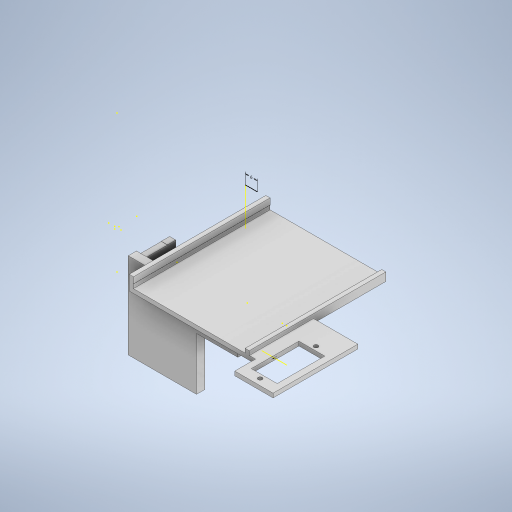
# Autodesk Inventor part: btholder
Saved by Autodesk Inventor 2023 (Build 270158000, 158)
## iProperties
Created: 2023-04-13
Part Number: btholder
Material: Generic
Document SubType Name: Modeling
Designer: Markus
Density: 1 g/cm^3
Appearance: Default
Author: Markus
Autodesk Inventor part; units mm, degrees
ref_plane "YZ Plane" through (0, 0, 0) normal (1, 0, 0) x (0, 1, 0)
ref_plane "XZ Plane" through (0, 0, 0) normal (0, 1, 0) x (-1, 0, 0)
ref_plane "XY Plane" through (0, 0, 0) normal (0, 0, 1) x (1, 0, 0)
sketch "Sketch1" plane through (0, 0, 0) normal (1, 0, 0) x (0, 1, 0)
  line L0 (0, 0) -> (20.5296, 0)
  line L1 (20.5296, -23) -> (0, -23)
  line L2 (0, -23) -> (0, 0)
  line L3 (0, 0) -> (50, 0)
  line L4 (50, 0) -> (50, -23)
  line L5 (50, -23) -> (0, -23)
  line L6 (0, -23) -> (0, 0)
  dimension "d0" = 23
  dimension "d1" = 50
  constraints: 14 end point, 3 parallel, 2 horizontal, 1 perpendicular, 1 point on line
  measures "d0" distance of L0.end L1.start
  measures "d1" distance of L4.end L5.end
extrude "Extrusion1" add sketch "Sketch1" along normal blind 2
sketch "Sketch2" plane through (2, 0, 0) normal (1, 0, 0) x (0, 0, -1)
  line L0 (23, 50) -> (0, 50) projected
  line L1 (13.5, 0) -> (9.5, 0)
  line L2 (9.5, 0) -> (9.5, 50)
  line L3 (9.5, 50) -> (13.5, 50)
  line L4 (13.5, 50) -> (13.5, 0)
  line L5 (13.5, 0) -> (9.5, 50) construction
  line L6 (9.5, 0) -> (13.5, 50) construction
  point P0 (0, 0)
  point P1 (17.2504, 25)
  point P2 (11.5, 25)
  dimension "d4" = 4
  constraints: 12 end point, 2 midpoint, 2 parallel, 1 horizontal, 1 perpendicular, 1 point on line
  measures "d4" distance of L2.end L3.end
sketch "Sketch3" plane through (0, 0, 0) normal (-1, 0, 0) x (0, 0, 1)
  line L0 (-23, 50) -> (0, 50) projected
  line L1 (-23, 50) -> (0, 50)
  line L2 (0, 50) -> (0, 0)
  line L3 (0, 0) -> (-23, 0)
  line L4 (-23, 0) -> (-23, 50)
  constraints: 8 end point, 2 parallel, 1 horizontal, 1 perpendicular
extrude "Extrusion2" add sketch "Sketch3" along normal blind 1
sketch "Sketch4" plane through (2, 0, 0) normal (1, 0, 0) x (0, 0, -1)
  point P0 (0, 0)
extrude "Extrusion3" add sketch "Sketch2" along normal blind 29
sketch "Sketch5" plane through (2, 0, -9.5) normal (0, 0, 1) x (1, 0, 0)
  line L0 (0, 50) -> (29, 50) projected
  line L1 (29, 0) -> (27, 0)
  line L2 (27, 0) -> (27, 50)
  line L3 (27, 50) -> (29, 50)
  line L4 (29, 50) -> (29, 0)
  point P0 (-2, 0)
  dimension "d9" = 2
  constraints: 8 end point, 2 parallel, 1 horizontal, 1 perpendicular, 1 point on line
  measures "d9" distance of L2.end L3.end
extrude "Extrusion4" add sketch "Sketch5" along normal blind 17.5
sketch "Sketch6" plane through (2, 0, -13.5) normal (0, 0, -1) x (-1, 0, 0)
  line L0 (-29, 50) -> (-27, 50) projected
  line L1 (-27, 50) -> (-27, 0) projected
  line L2 (-29, 50) -> (-27, 50)
  line L3 (-27, 50) -> (-27, 0)
  line L4 (-27, 0) -> (-29, 0)
  line L5 (-29, 0) -> (-29, 50)
  point P0 (2, 0)
  constraints: 8 end point, 2 parallel, 1 horizontal, 1 perpendicular
extrude "Extrusion5" add sketch "Sketch6" along normal blind 17.5
sketch "Sketch7" plane through (31, 0, 0) normal (1, 0, 0) x (0, 0, -1)
  line L0 (-8, 0) -> (-8, 50) projected
  line L1 (31, 50) -> (31, 0) projected
  line L2 (-8, 50) -> (31, 50)
  line L3 (31, 50) -> (31, 48)
  line L4 (31, 48) -> (-8, 48)
  line L5 (-8, 48) -> (-8, 50)
  point P0 (0, 0)
  dimension "d14" = 2
  constraints: 8 end point, 2 parallel, 1 horizontal, 1 perpendicular, 1 point on line
  measures "d14" distance of L2.end L3.end
extrude "Extrusion6" add sketch "Sketch7" along normal blind 32
sketch "Sketch8" plane through (31, 48, -31) normal (0, -1, 0) x (1, 0, 0)
  line L0 (32, 39) -> (32, 0) projected
  line L1 (0, 0) -> (32, 0) projected
  line L2 (32, 39) -> (30, 39)
  line L3 (30, 39) -> (30, 0)
  line L4 (30, 0) -> (32, 0)
  line L5 (32, 0) -> (32, 39)
  point P0 (-31, 31)
  dimension "d17" = 2
  constraints: 8 end point, 2 parallel, 1 horizontal, 1 perpendicular, 1 point on line
  measures "d17" distance of L4.end L3.end
extrude "Extrusion7" add sketch "Sketch8" along normal up to surface (48 mm away)
sketch "Sketch9" plane through (31, 48, -31) normal (0, -1, 0) x (1, 0, 0)
  point P0 (-31, 31)
sketch "Sketch10" plane through (61, 0, 8) normal (0, -1, 0) x (1, 0, 0)
  line L0 (2, -39) -> (2, 0) projected
  line L1 (-32, -17.5) -> (-32, 0) projected
  line L2 (2, 0) -> (-32, 0)
  line L3 (-32, 0) -> (-32, -9)
  line L4 (-32, -9) -> (2, -9)
  line L5 (2, -9) -> (2, 0)
  point P0 (-61, -8)
  dimension "d20" = 9
  constraints: 8 end point, 2 parallel, 1 horizontal, 1 perpendicular, 1 point on line
  measures "d20" distance of L3.end L2.end
extrude "Extrusion8" cut sketch "Sketch10" against normal blind 50
sketch "Sketch11" plane through (2, 0, -31) normal (0, 0, -1) x (-1, 0, 0)
  line L0 (-61, 50) -> (-61, 0) projected
  line L1 (0, 50) -> (-27, 50) projected
  line L2 (-61, 0) -> (-27, 0)
  line L3 (-27, 0) -> (-27, 50)
  line L4 (-27, 50) -> (-61, 50)
  line L5 (-61, 50) -> (-61, 0)
  point P0 (2, 0)
  constraints: 8 end point, 2 parallel, 1 horizontal, 1 perpendicular
extrude "Extrusion9" add sketch "Sketch11" along normal blind 2
sketch "Sketch12" plane through (-1, 0, 0) normal (0, -1, 0) x (1, 0, 0)
  line L0 (62, -1) -> (32, -1) projected
  line L1 (64, -1) -> (64, -33) projected
  line L2 (62, -1) -> (64, -1)
  line L3 (64, -1) -> (64, -31.0308)
  line L4 (64, -31.0308) -> (62, -31.0308)
  line L5 (62, -31.0308) -> (62, -1)
  point P0 (1, 0)
  constraints: 8 end point, 2 parallel, 1 horizontal, 1 perpendicular, 1 point on line
extrude "Extrusion10" add sketch "Sketch12" along normal blind 20.5
sketch "Sketch13" plane through (61, 48, -31) normal (-1, 0, 0) x (0, 0, 1)
  line L0 (30, -68.5) -> (-0.0308, -68.5) projected
  line L1 (30, 0) -> (30, -68.5) projected
  line L2 (-0.0308, -68.5) -> (30, -68.5)
  line L3 (30, -68.5) -> (30, -66.5)
  line L4 (30, -66.5) -> (-0.0308, -66.5)
  line L5 (-0.0308, -66.5) -> (-0.0308, -68.5)
  point P0 (31, -48)
  dimension "d27" = 2
  constraints: 8 end point, 2 parallel, 1 horizontal, 1 perpendicular, 1 point on line
  measures "d27" distance of L3.end L2.end
extrude "Extrusion11" add sketch "Sketch13" along normal up to surface (32 mm away)
sketch "Sketch14" plane through (-1, 0, 0) normal (0, -1, 0) x (1, 0, 0)
  line L0 (64, -33) -> (30, -33) projected
  line L1 (64, -31.0308) -> (30, -31.0308) projected
  line L2 (64, -33) -> (30, -33)
  line L3 (30, -33) -> (30, -31.0308)
  line L4 (30, -31.0308) -> (64, -31.0308)
  line L5 (64, -31.0308) -> (64, -33)
  point P0 (1, 0)
  point P1 (30, -33)
  constraints: 8 end point, 2 parallel, 1 horizontal, 1 perpendicular
extrude "Extrusion12" add sketch "Sketch14" along normal up to surface (20.5 mm away)
sketch "Sketch15" plane through (61, 48, -31) normal (-1, 0, 0) x (0, 0, 1)
  line L0 (-0.0308, -66.5) -> (30, -66.5) projected
  line L1 (30, 0) -> (30, -66.5) projected
  line L2 (-0.0308, -66.5) -> (30, -66.5)
  line L3 (30, -66.5) -> (30, -48)
  line L4 (30, -48) -> (-0.0308, -48)
  line L5 (-0.0308, -48) -> (-0.0308, -66.5)
  point P0 (31, -48)
  constraints: 8 end point, 2 parallel, 1 horizontal, 1 perpendicular, 1 point on line
extrude "Extrusion13" cut sketch "Sketch15" against normal blind 10
sketch "Sketch16" plane through (-1, 0, 0) normal (0, -1, 0) x (1, 0, 0)
  line L0 (32, -31) -> (32, -1) projected
  line L1 (30, -33) -> (64, -33) projected
  line L2 (32, -1) -> (30, -1)
  line L3 (30, -1) -> (30, -33)
  line L4 (30, -33) -> (32, -33)
  line L5 (32, -33) -> (32, -1)
  point P0 (1, 0)
  constraints: 8 end point, 2 parallel, 1 horizontal, 1 perpendicular
extrude "Extrusion14" add sketch "Sketch16" along normal up to surface (18.5 mm away)
sketch "Sketch17" plane through (31, 0, -31.0308) normal (0, 0, 1) x (1, 0, 0)
  line L0 (0, 48) -> (0, -18.5) projected
  line L1 (32, 50) -> (32, -20.5) projected
  line L2 (0, -18.5) -> (32, -18.5)
  line L3 (32, -18.5) -> (32, 0)
  line L4 (32, 0) -> (0, 0)
  line L5 (0, 0) -> (0, -18.5)
  point P0 (-31, 0)
  constraints: 8 end point, 2 parallel, 1 horizontal, 1 perpendicular, 1 point on line
extrude "Extrusion15" cut sketch "Sketch17" against normal blind 10
sketch "Sketch18" plane through (31, 0, 0) normal (1, 0, 0) x (0, 0, -1)
  line L0 (1, 48) -> (1, -18.5) projected
  line L1 (31, 0) -> (1, 0) projected
  line L2 (1, -18.5) -> (3, -18.5)
  line L3 (3, -18.5) -> (3, 0)
  line L4 (3, 0) -> (1, 0)
  line L5 (1, 0) -> (1, -18.5)
  point P0 (0, 0)
  dimension "d38" = 2
  constraints: 8 end point, 2 parallel, 1 horizontal, 1 perpendicular, 1 point on line
  measures "d38" distance of L4.end L3.end
extrude "Extrusion16" add sketch "Sketch18" along normal blind 13
sketch "Sketch19" plane through (29, 50, -1) normal (0, 0, 1) x (1, 0, 0)
  line L0 (34, -68.5) -> (34, -70.5) projected
  line L1 (34, -70.5) -> (0, -70.5) projected
  line L2 (34, -68.5) -> (0, -68.5)
  line L3 (0, -68.5) -> (0, -70.5)
  line L4 (0, -70.5) -> (34, -70.5)
  line L5 (34, -70.5) -> (34, -68.5)
  point P0 (-29, -50)
  constraints: 8 end point, 2 parallel, 1 horizontal, 1 perpendicular
extrude "Extrusion17" add sketch "Sketch19" along normal blind 2
sketch "Sketch20" plane through (31, -18.5, -33) normal (0, 1, 0) x (1, 0, 0)
  point P0 (-31, -33)
sketch "Sketch21" plane through (29, 50, -1) normal (0, 0, 1) x (1, 0, 0)
  line L0 (15, -50) -> (15, -68.5) projected
  line L1 (2, -68.5) -> (15, -68.5) projected
  line L2 (15, -50) -> (2, -50)
  line L3 (2, -50) -> (2, -68.5)
  line L4 (2, -68.5) -> (15, -68.5)
  line L5 (15, -68.5) -> (15, -50)
  point P0 (-29, -50)
  constraints: 8 end point, 2 parallel, 1 horizontal, 1 perpendicular
extrude "Extrusion18" cut sketch "Sketch21" against normal blind 2
sketch "Sketch22" plane through (31, -18.5, -33) normal (0, 1, 0) x (1, 0, 0)
  line L0 (32, -34) -> (-2, -34) projected
  line L1 (30, -32) -> (0, -32) projected
  line L2 (-2, -34) -> (13, -34)
  line L3 (13, -34) -> (13, -32)
  line L4 (13, -32) -> (-2, -32)
  line L5 (-2, -32) -> (-2, -34)
  point P0 (-31, -33)
  dimension "d45" = 15
  constraints: 8 end point, 2 parallel, 1 horizontal, 1 perpendicular, 1 point on line
  measures "d45" distance of L4.end L3.end
extrude "Extrusion19" add sketch "Sketch22" along normal blind 4
sketch "Sketch23" plane through (29, 50, 1) normal (0, 0, 1) x (1, 0, 0)
  point P0 (-29, -50)
sketch "Sketch24" plane through (63, 0, 0) normal (1, 0, 0) x (0, 0, -1)
  point P0 (0, 0)
sketch "Sketch25" plane through (63, 0, 0) normal (1, 0, 0) x (0, 0, -1)
  line L0 (-1, -20.5) -> (-1, -18.5) projected
  line L1 (33, -20.5) -> (-1, -20.5) projected
  line L2 (-1, -18.5) -> (33, -18.5)
  line L3 (33, -18.5) -> (33, -20.5)
  line L4 (33, -20.5) -> (-1, -20.5)
  line L5 (-1, -20.5) -> (-1, -18.5)
  point P0 (0, 0)
  constraints: 8 end point, 2 parallel, 1 horizontal, 1 perpendicular
extrude "Extrusion20" add sketch "Sketch25" along normal blind 5
sketch "Sketch26" plane through (68, 0, 0) normal (1, 0, 0) x (0, 0, -1)
  line L0 (1, -18.5) -> (33, -18.5) projected
  line L1 (33, -20.5) -> (-1, -20.5) projected
  line L2 (2.0812, -18.5) -> (-1, -18.5)
  line L3 (-1, -18.5) -> (-1, -20.5)
  line L4 (-1, -20.5) -> (2.0812, -20.5)
  line L5 (2.0812, -20.5) -> (2.0812, -18.5)
  point P0 (0, 0)
  constraints: 8 end point, 2 parallel, 1 horizontal, 1 perpendicular, 1 point on line
extrude "Extrusion21" add sketch "Sketch26" along normal blind 14
sketch "Sketch27" plane through (68, -20.5, -2.0812) normal (0, 0, -1) x (-1, 0, 0)
  line L0 (-14, 2) -> (-14, 0) projected
  line L1 (39, 0) -> (-14, 0) projected
  line L2 (-14, 2) -> (-12, 2)
  line L3 (-12, 2) -> (-12, 0)
  line L4 (-12, 0) -> (-14, 0)
  line L5 (-14, 0) -> (-14, 2)
  point P0 (68, 20.5)
  dimension "d52" = 2
  constraints: 8 end point, 2 parallel, 1 horizontal, 1 perpendicular, 1 point on line
  measures "d52" distance of L3.end L4.end
extrude "Extrusion22" add sketch "Sketch27" along normal blind 25
sketch "Sketch28" plane through (80, -20.5, -2.0812) normal (-1, 0, 0) x (0, 0, 1)
  point P0 (2.0812, 20.5)
sketch "Sketch29" plane through (80, -20.5, -2.0812) normal (-1, 0, 0) x (0, 0, 1)
  line L0 (-25, 2) -> (-25, 0) projected
  line L1 (3.0812, 0) -> (-25, 0) projected
  line L2 (-25, 2) -> (-23, 2)
  line L3 (-23, 2) -> (-23, 0)
  line L4 (-23, 0) -> (-25, 0)
  line L5 (-25, 0) -> (-25, 2)
  point P0 (2.0812, 20.5)
  dimension "d55" = 2
  constraints: 8 end point, 2 parallel, 1 horizontal, 1 perpendicular, 1 point on line
  measures "d55" distance of L3.end L4.end
extrude "Extrusion23" add sketch "Sketch29" along normal up to surface (12 mm away)
sketch "Sketch30" plane through (68, -20.5, -27.0812) normal (0, 0, -1) x (-1, 0, 0)
  line L0 (-14, 2) -> (-14, 0) projected
  line L1 (0, 0) -> (-12, 0) projected
  line L2 (-14, 2) -> (0, 2)
  line L3 (0, 2) -> (0, 0)
  line L4 (0, 0) -> (-14, 0)
  line L5 (-14, 0) -> (-14, 2)
  point P0 (68, 20.5)
  constraints: 8 end point, 2 parallel, 1 horizontal, 1 perpendicular
extrude "Extrusion24" add sketch "Sketch30" along normal up to surface (5.9188 mm away)
sketch "Sketch31" plane through (31, -18.5, -1) normal (0, 1, 0) x (1, 0, 0)
  line L0 (37, 1.0812) -> (49, 1.0812) projected
  line L1 (43, 1.0812) -> (43, 0.2954)
  point P0 (-31, -1)
  constraints: 2 end point, 1 midpoint, 1 vertical
sketch "Sketch32" plane through (29, 50, 1) normal (0, 0, 1) x (1, 0, 0)
  line L0 (53, -68.5) -> (53, -70.5) projected
  line L1 (15, -68.5) -> (53, -68.5) projected
  line L2 (53, -70.5) -> (15, -70.5)
  line L3 (15, -70.5) -> (15, -68.5)
  line L4 (15, -68.5) -> (53, -68.5)
  line L5 (53, -68.5) -> (53, -70.5)
  point P0 (-29, -50)
  constraints: 8 end point, 2 parallel, 1 horizontal, 1 perpendicular
extrude "Extrusion25" add sketch "Sketch32" along normal blind 2
sketch "Sketch33" plane through (31, -18.5, -1) normal (0, 1, 0) x (1, 0, 0)
  line L0 (37, 1.0812) -> (49, 1.0812) projected
  circle A0 centre (43, -0.9188) radius 1
  line L1 (49, 24.0812) -> (37, 24.0812) projected
  circle A1 centre (43, 26.0812) radius 1
  point P0 (-31, -1)
  dimension "d63" = 2
  constraints: 2 centre point
  measures "d63" diameter of A0
extrude "Extrusion26" cut sketch "Sketch33" against normal blind 5
thread "Thread1" size "M2x0.4" class "6H" standard "ANSI Metric M Profile" full length
thread "Thread2" size "M2x0.4" class "6H" standard "ANSI Metric M Profile" full length
sketch "Sketch34" plane through (2, 0, -33) normal (0, 0, -1) x (-1, 0, 0)
  line L0 (-27, 50) -> (-27, -20.5) projected
  line L1 (-80, -18.5) -> (-42, -18.5) projected
  line L2 (-27, -20.5) -> (-61, -20.5)
  line L3 (-61, -20.5) -> (-61, -18.5)
  line L4 (-61, -18.5) -> (-27, -18.5)
  line L5 (-27, -18.5) -> (-27, -20.5)
  point P0 (2, 0)
  point P1 (-42, -18.5)
  constraints: 8 end point, 2 parallel, 1 horizontal, 1 midpoint, 1 perpendicular
extrude "Extrusion27" add sketch "Sketch34" along normal blind 30
sketch "Sketch35" plane through (31, -18.5, -1) normal (0, 1, 0) x (1, 0, 0)
  line L0 (0, 0) -> (0, 32) projected
  line L1 (-2, 62) -> (-2, -2) projected
  line L2 (0, 32) -> (-2, 32)
  line L3 (-2, 32) -> (-2, 62)
  line L4 (-2, 62) -> (0, 62)
  line L5 (0, 62) -> (0, 32)
  point P0 (-31, -1)
  constraints: 8 end point, 2 parallel, 1 horizontal, 1 perpendicular
extrude "Extrusion28" add sketch "Sketch35" along normal blind 2
sketch "Sketch36" plane through (63, -20.5, -33) normal (1, 0, 0) x (0, 0, -1)
  line L0 (0, 0) -> (0, 2) projected
  line L1 (0, 2) -> (30, 2)
  line L2 (30, 2) -> (30, 0)
  line L3 (30, 0) -> (0, 0)
  line L4 (0, 0) -> (0, 2)
  point P0 (-33, 20.5)
  constraints: 8 end point, 2 parallel, 1 horizontal, 1 perpendicular
extrude "Extrusion29" add sketch "Sketch36" along normal blind 4
sketch "Sketch37" plane through (31, -18.5, -1) normal (0, 1, 0) x (1, 0, 0)
  line L0 (0, 62) -> (36, 62) projected
  line L1 (51, -4) -> (13, -4) projected
  line L2 (36, 62) -> (34, 62)
  line L3 (34, 62) -> (34, -4)
  line L4 (34, -4) -> (36, -4)
  line L5 (36, -4) -> (36, 62)
  point P0 (-31, -1)
  dimension "d77" = 2
  constraints: 8 end point, 2 parallel, 1 horizontal, 1 perpendicular, 1 point on line
  measures "d77" distance of L4.end L3.end
extrude "Extrusion30" add sketch "Sketch37" along normal blind 2
sketch "Sketch38" plane through (29, 50, -1) normal (0, 0, 1) x (1, 0, 0)
  line L0 (2, -2) -> (2, -64.5) projected
  line L1 (0, 0) -> (0, -66.5) projected
  line L2 (2, -2) -> (0, -2)
  line L3 (0, -2) -> (0, -20)
  line L4 (0, -20) -> (2, -20)
  line L5 (2, -20) -> (2, -2)
  line L6 (34, -50) -> (2, -50) projected
  line L7 (0, -20) -> (34, -20)
  line L8 (34, -20) -> (34, -50)
  line L9 (34, -50) -> (0, -50)
  line L10 (0, -50) -> (0, -20)
  point P0 (-29, -50)
  dimension "d80" = 18
  constraints: 16 end point, 4 parallel, 2 horizontal, 2 perpendicular, 1 point on line
  measures "d80" distance of L3.end L2.end
extrude "Extrusion31" add sketch "Sketch38" along normal blind 2 contours L7 L8 L6 L0
sketch "Sketch39" plane through (29, 50, -1) normal (0, 0, 1) x (1, 0, 0)
  line L0 (-27, -50) -> (0, -50) projected
  line L1 (2, -20) -> (2, -50) projected
  line L2 (0, -50) -> (2, -50)
  line L3 (2, -50) -> (2, -20)
  line L4 (2, -20) -> (0, -20)
  line L5 (0, -20) -> (0, -50)
  point P0 (-29, -50)
  constraints: 8 end point, 2 parallel, 1 horizontal, 1 perpendicular
extrude "Extrusion32" add sketch "Sketch39" along normal blind 2
sketch "Sketch40" plane through (29, 50, 1) normal (0, 0, 1) x (1, 0, 0)
  line L0 (34, -50) -> (34, -20) projected
  line L1 (0, -20) -> (34, -20)
  line L2 (34, -20) -> (34, -20.389)
  line L3 (34, -20.389) -> (0, -20.389)
  line L4 (0, -20.389) -> (0, -20)
  point P0 (-29, -50)
  dimension "d85" = 0.389
  constraints: 8 end point, 2 parallel, 1 horizontal, 1 perpendicular, 1 point on line
  measures "d85" distance of L1.end L2.end
extrude "Extrusion33" cut sketch "Sketch40" against normal blind 2
sketch "Sketch41" plane through (29, 50, 1) normal (0, 0, 1) x (1, 0, 0)
  point P0 (-29, -50)
sketch "Sketch42" plane through (29, 50, -1) normal (0, 0, 1) x (1, 0, 0)
  line L0 (32, -2) -> (32, -20.389) projected
  line L1 (32, -2) -> (38, -2)
  point P0 (-29, -50)
  dimension "d88" = 6
  constraints: 2 end point, 1 horizontal
  measures "d88" distance of L0.start L1.end
sketch "Sketch43" plane through (63, 0, 0) normal (1, 0, 0) x (0, 0, -1)
  line L0 (9.5, 50) -> (1, 50) projected
  line L1 (31, 48) -> (1, 48) projected
  line L2 (1, 50) -> (31, 50)
  line L3 (31, 50) -> (31, 48)
  line L4 (31, 48) -> (1, 48)
  line L5 (1, 48) -> (1, 50)
  point P0 (0, 0)
  point P1 (1, 48)
  constraints: 8 end point, 2 parallel, 1 horizontal, 1 perpendicular
extrude "Extrusion34" add sketch "Sketch43" along normal blind 6
sketch "Sketch44" plane through (63, 0, 0) normal (1, 0, 0) x (0, 0, -1)
  line L0 (33, 50) -> (33, 0) projected
  line L1 (31, 0) -> (33, 0) projected
  line L2 (33, 50) -> (31, 50)
  line L3 (31, 50) -> (31, 0)
  line L4 (31, 0) -> (33, 0)
  line L5 (33, 0) -> (33, 50)
  point P0 (0, 0)
  constraints: 8 end point, 2 parallel, 1 horizontal, 1 perpendicular
extrude "Extrusion35" add sketch "Sketch44" along normal blind 6
sketch "Sketch45" plane through (63, 0, 0) normal (1, 0, 0) x (0, 0, -1)
  point P0 (0, 0)
sketch "Sketch46" plane through (63, 0, 0) normal (1, 0, 0) x (0, 0, -1)
  line L0 (-1, 0) -> (-1, 29.611) projected
  line L1 (31, 0) -> (31, 48) projected
  line L2 (-1, 0) -> (31, 0)
  line L3 (31, 0) -> (31, 2)
  line L4 (31, 2) -> (-1, 2)
  line L5 (-1, 2) -> (-1, 0)
  point P0 (0, 0)
  point P1 (-1, 2)
  dimension "d93" = 2
  constraints: 8 end point, 2 parallel, 1 horizontal, 1 perpendicular, 1 point on line
  measures "d93" distance of L3.end L2.end
extrude "Extrusion36" add sketch "Sketch46" along normal blind 6
sketch "Sketch47" plane through (63, 48, -31) normal (0, 0, 1) x (1, 0, 0)
  line L0 (0, 0) -> (6, 0) projected
  line L1 (0, -46) -> (6, -46) projected
  line L2 (6, 0) -> (4, 0)
  line L3 (4, 0) -> (4, -46)
  line L4 (4, -46) -> (6, -46)
  line L5 (6, -46) -> (6, 0)
  point P0 (-63, -48)
  point P1 (4, 0)
  dimension "d96" = 2
  constraints: 8 end point, 2 parallel, 1 horizontal, 1 perpendicular, 1 point on line
  measures "d96" distance of L4.end L3.end
sketch "Sketch48" plane through (63, 0, 0) normal (1, 0, 0) x (0, 0, -1)
  line L0 (31, 48) -> (1, 48) projected
  line L1 (1, 48) -> (31, 48)
  line L2 (31, 48) -> (31, 2)
  line L3 (31, 2) -> (1, 2)
  line L4 (1, 2) -> (1, 48)
  point P0 (0, 0)
  constraints: 8 end point, 2 parallel, 1 horizontal, 1 perpendicular
extrude "Extrusion37" cut sketch "Sketch48" against normal blind 10
extrude "Extrusion38" add sketch "Sketch47" along normal up to surface (30 mm away)
sketch "Sketch49" plane through (63, 0, 0) normal (1, 0, 0) x (0, 0, -1)
  line L0 (1, 2) -> (1, 0) projected
  line L1 (-1, 29.611) -> (1, 29.611)
  line L2 (1, 29.611) -> (1, 2)
  line L3 (1, 2) -> (-1, 2)
  line L4 (-1, 2) -> (-1, 29.611)
  point P0 (0, 0)
  constraints: 8 end point, 2 parallel, 1 horizontal, 1 perpendicular
extrude "Extrusion39" add sketch "Sketch49" along normal up to surface (6 mm away)
sketch "Sketch50" plane through (31, 0, -31) normal (0, -1, 0) x (1, 0, 0)
  line L0 (0, 30) -> (30, 30) projected
  line L1 (36, 30) -> (36, 0) projected
  line L2 (30, 30) -> (36, 30)
  line L3 (36, 30) -> (36, 0)
  line L4 (36, 0) -> (30, 0)
  line L5 (30, 0) -> (30, 30)
  point P0 (-31, 31)
  constraints: 8 end point, 2 parallel, 1 horizontal, 1 perpendicular
extrude "Extrusion40" cut sketch "Sketch50" against normal blind 10
sketch "Sketch51" plane through (-1, 0, 0) normal (-1, 0, 0) x (0, 0, 1)
  line L0 (-23, 0) -> (-23, 50) projected
  line L1 (-23, 0) -> (0, 0)
  line L2 (0, 0) -> (0, 50)
  line L3 (0, 50) -> (-23, 50)
  line L4 (-23, 50) -> (-23, 0)
  constraints: 8 end point, 2 parallel, 1 horizontal, 1 perpendicular
extrude "Extrusion41" cut sketch "Sketch51" against normal blind 3
sketch "Sketch52" plane through (29, 0, -9.5) normal (0, 0, 1) x (1, 0, 0)
  point P0 (-29, 0)
sketch "Sketch53" plane through (2, 0, 0) normal (-1, 0, 0) x (0, 0, 1)
  line L0 (-13.5, 50) -> (-13.5, 0) projected
  line L1 (-9.5, 0) -> (-9.5, 50) projected
  line L2 (-13.5, 50) -> (-9.5, 50)
  line L3 (-9.5, 50) -> (-9.5, 0)
  line L4 (-9.5, 0) -> (-13.5, 0)
  line L5 (-13.5, 0) -> (-13.5, 50)
  point P0 (0, 0)
  constraints: 8 end point, 2 parallel, 1 horizontal, 1 perpendicular
extrude "Extrusion42" add sketch "Sketch53" along normal blind 6
sketch "Sketch54" plane through (29, 0, -9.5) normal (0, 0, 1) x (1, 0, 0)
  line L0 (0, 50) -> (-33, 50) projected
  line L1 (-33, 0) -> (0, 0) projected
  line L2 (-33, 50) -> (-30, 50)
  line L3 (-30, 50) -> (-30, 0)
  line L4 (-30, 0) -> (-33, 0)
  line L5 (-33, 0) -> (-33, 50)
  point P0 (-29, 0)
  dimension "d109" = 3
  constraints: 8 end point, 2 parallel, 1 horizontal, 1 perpendicular, 1 point on line
  measures "d109" distance of L3.end L4.end
sketch "Sketch55" plane through (29, 0, -13.5) normal (0, 0, -1) x (-1, 0, 0)
  line L0 (33, 50) -> (33, 0) projected
  line L1 (33, 0) -> (0, 0) projected
  line L2 (33, 50) -> (30, 50)
  line L3 (30, 50) -> (30, 0)
  line L4 (30, 0) -> (33, 0)
  line L5 (33, 0) -> (33, 50)
  point P0 (29, 0)
  dimension "d110" = 3
  constraints: 8 end point, 2 parallel, 1 horizontal, 1 perpendicular, 1 point on line
  measures "d110" distance of L4.end L3.end
extrude "Extrusion43" add sketch "Sketch55" along normal blind 12
sketch "Sketch56" plane through (29, 0, -13.5) normal (0, -1, 0) x (1, 0, 0)
  line L0 (-33, 4) -> (-33, -12) projected
  line L1 (0, 4) -> (-33, 4) projected
  line L2 (-33, -12) -> (-30.0022, -12)
  line L3 (-30.0022, -12) -> (-30.0022, 4)
  line L4 (-30.0022, 4) -> (-33, 4)
  line L5 (-33, 4) -> (-33, -12)
  line L6 (-30, 0) -> (0, 0) projected
  line L7 (-30.0022, 4) -> (0, 4)
  line L8 (0, 4) -> (0, 0)
  line L9 (0, 0) -> (-30.0022, 0)
  line L10 (-30.0022, 0) -> (-30.0022, 4)
  point P0 (-29, 13.5)
  constraints: 16 end point, 4 parallel, 2 horizontal, 2 perpendicular, 1 point on line
extrude "Extrusion44" add sketch "Sketch56" along normal blind 60
sketch "Sketch57" plane through (29, 50, 1) normal (0, 0, 1) x (1, 0, 0)
  point P0 (-29, -50)
sketch "Sketch58" plane through (-4, 0, 0) normal (-1, 0, 0) x (0, 0, 1)
  point P0 (0, 0)
sketch "Sketch59" plane through (-4, 0, 0) normal (-1, 0, 0) x (0, 0, 1)
  point P0 (0, 0)
extrude "Extrusion45" cut sketch "Sketch54" against normal blind 50
sketch "Sketch60" plane through (-1, 0, -9.5) normal (-1, 0, 0) x (0, 0, 1)
  line L0 (-4, 0) -> (-4, 50) projected
  line L1 (0, 0) -> (0, -60) projected
  line L2 (-4, 50) -> (0, 50)
  line L3 (0, 50) -> (0, 0)
  line L4 (0, 0) -> (-4, 0)
  line L5 (-4, 0) -> (-4, 50)
  point P0 (9.5, 0)
  constraints: 8 end point, 2 parallel, 1 horizontal, 1 perpendicular
extrude "Extrusion46" cut sketch "Sketch60" against normal up to surface (30 mm away)
sketch "Sketch61" plane through (29, -60, -9.5) normal (1, 0, 0) x (0, 0, -1)
  point P0 (-9.5, 60)
sketch "Sketch62" plane through (-4, 0, 0) normal (-1, 0, 0) x (0, 0, 1)
  line L0 (-63, -20.5) -> (-13.5, -20.5) projected
  line L1 (-13.5, 0) -> (-25.5, 0) projected
  line L2 (-25.4638, -20.5) -> (-13.5, -20.5)
  line L3 (-13.5, -20.5) -> (-13.5, 0)
  line L4 (-13.5, 0) -> (-25.4638, 0)
  line L5 (-25.4638, 0) -> (-25.4638, -20.5)
  point P0 (0, 0)
  point P1 (-13.5, -20.5)
  constraints: 8 end point, 2 parallel, 1 horizontal, 1 perpendicular, 1 point on line
extrude "Extrusion47" cut sketch "Sketch62" against normal blind 10
sketch "Sketch63" plane through (29, 0, -25.5) normal (0, 0, -1) x (-1, 0, 0)
  line L0 (33, 0) -> (30.0022, 0) projected
  line L1 (30.0022, 0) -> (30.0022, -20.5) projected
  line L2 (33, 0) -> (30.0022, 0)
  line L3 (30.0022, 0) -> (30.0022, -20.5)
  line L4 (30.0022, -20.5) -> (33, -20.5)
  line L5 (33, -20.5) -> (33, 0)
  point P0 (29, 0)
  constraints: 8 end point, 2 parallel, 1 horizontal, 1 perpendicular
extrude "Extrusion48" cut sketch "Sketch63" against normal blind 2
sketch "Sketch64" plane through (29, 0, -25.5) normal (0, 0, -1) x (-1, 0, 0)
  line L0 (30.0022, -20.5) -> (30.0022, -60) projected
  line L1 (33, 0) -> (33, -60) projected
  line L2 (30.0022, -60) -> (33, -60)
  line L3 (33, -60) -> (33, -20.4178)
  line L4 (33, -20.4178) -> (30.0022, -20.4178)
  line L5 (30.0022, -20.4178) -> (30.0022, -60)
  point P0 (29, 0)
  constraints: 8 end point, 2 parallel, 1 horizontal, 1 perpendicular, 1 point on line
extrude "Extrusion49" add sketch "Sketch64" along normal blind 4
sketch "Sketch65" plane through (-1.0022, -60, -13.5) normal (1, 0, 0) x (0, 0, -1)
  point P0 (-13.5, 60)
sketch "Sketch66" plane through (-1.0022, -60, -13.5) normal (1, 0, 0) x (0, 0, -1)
  line L0 (16, 0) -> (16, 39.5822) projected
  line L1 (16, 19.7911) -> (8, 19.7911)
  circle A0 centre (8, 19.7911) radius 2
  circle A1 centre (8, 31.9197) radius 2
  circle A2 centre (8, 5.9419) radius 2
  point P0 (-13.5, 60)
  dimension "d125" = 8
  dimension "d126" = 4
  dimension "d127" = 4
  dimension "d128" = 4
  constraints: 3 centre point, 2 end point, 1 coincident, 1 horizontal, 1 midpoint
  measures "d125" distance of L1.start L1.end
  measures "d126" diameter of A0
  measures "d127" diameter of A1
  measures "d128" diameter of A2
extrude "Extrusion50" cut sketch "Sketch66" against normal blind 4
sketch "Sketch67" plane through (69, 0, 0) normal (1, 0, 0) x (0, 0, -1)
  line L0 (1, 0) -> (-1, 0) projected
  line L1 (-1, 0) -> (33, 0)
  line L2 (33, 0) -> (33, 52.0409)
  line L3 (33, 52.0409) -> (-1, 52.0409)
  line L4 (-1, 52.0409) -> (-1, 0)
  point P0 (0, 0)
  constraints: 8 end point, 2 parallel, 1 horizontal, 1 perpendicular
extrude "Extrusion51" cut sketch "Sketch67" against normal up to surface (40 mm away)
sketch "Sketch68" plane through (29, -60, -9.5) normal (1, 0, 0) x (0, 0, -1)
  line L0 (0, 60) -> (0, 0) projected
  line L1 (4, 39.5) -> (4, 0) projected
  line L2 (0, 25.4882) -> (4, 25.4882)
  line L3 (4, 25.4882) -> (4, 39.5)
  line L4 (4, 39.5) -> (0, 39.5)
  line L5 (0, 39.5) -> (0, 25.4882)
  point P0 (-9.5, 60)
  constraints: 8 end point, 2 parallel, 1 horizontal, 1 perpendicular, 1 point on line
extrude "Extrusion52" add sketch "Sketch68" along normal blind 20
sketch "Sketch69" plane through (44, -18.5, -1) normal (1, 0, 0) x (0, 0, -1)
  line L0 (-2, 4) -> (0, 4) projected
  line L1 (0, 0) -> (0, 4) projected
  line L2 (-2, 4) -> (0, 4)
  line L3 (0, 4) -> (0, 0)
  line L4 (0, 0) -> (-2, 0)
  line L5 (-2, 0) -> (-2, 4)
  point P0 (-1, 18.5)
  constraints: 8 end point, 2 parallel, 1 horizontal, 1 perpendicular
extrude "Extrusion53" cut sketch "Sketch69" against normal blind 20
sketch "Sketch70" plane through (44, -20.5, 1) normal (-1, 0, 0) x (0, 0, 1)
  line L0 (0, 2) -> (-2, 2) projected
  line L1 (0, 2) -> (2, 2)
  line L2 (2, 2) -> (2, 0)
  line L3 (2, 0) -> (0, 0)
  line L4 (0, 0) -> (0, 2)
  point P0 (-1, 20.5)
  constraints: 8 end point, 2 parallel, 1 horizontal, 1 perpendicular
extrude "Extrusion54" add sketch "Sketch70" along normal up to surface (15 mm away)
sketch "Sketch71" plane through (31, 0, 0) normal (1, 0, 0) x (0, 0, -1)
  line L0 (1, 0) -> (9.5, 0) projected
  line L1 (33, -20.5) -> (33, -18.5) projected
  line L2 (1, 0) -> (33, 0)
  line L3 (33, 0) -> (33, -18.5)
  line L4 (33, -18.5) -> (1, -18.5)
  line L5 (1, -18.5) -> (1, 0)
  point P0 (0, 0)
  constraints: 8 end point, 2 parallel, 1 horizontal, 1 perpendicular
extrude "Extrusion55" cut sketch "Sketch71" against normal up to surface (35 mm away)
sketch "Sketch72" plane through (31, 0, 0) normal (1, 0, 0) x (0, 0, -1)
  line L0 (33, -16.5) -> (33, -18.5) projected
  line L1 (63, -20.5) -> (63, -16.5) projected
  line L2 (33, -16.5) -> (63, -16.5)
  line L3 (63, -16.5) -> (63, -18.5)
  line L4 (63, -18.5) -> (33, -18.5)
  line L5 (33, -18.5) -> (33, -16.5)
  point P0 (0, 0)
  constraints: 8 end point, 2 parallel, 1 horizontal, 1 midpoint, 1 perpendicular
extrude "Extrusion56" cut sketch "Sketch72" against normal blind 10
sketch "Sketch73" plane through (29, -20.5, -13.5) normal (-1, 0, 0) x (0, 0, 1)
  point P0 (13.5, 20.5)
sketch "Sketch74" plane through (29, -20.5, -13.5) normal (-1, 0, 0) x (0, 0, 1)
  line L0 (16.5, 2) -> (-49.5, 2) projected
  line L1 (4, 0) -> (0, 0) projected
  line L2 (-49.5, 2) -> (0, 2)
  line L3 (0, 2) -> (0, 0)
  line L4 (0, 0) -> (-49.5, 0)
  line L5 (-49.5, 0) -> (-49.5, 2)
  line L6 (16.5, 2) -> (4, 2) projected
  line L7 (4, 0) -> (16.5, 0) projected
  line L8 (4, 2) -> (16.5, 2)
  line L9 (16.5, 2) -> (16.5, 0)
  line L10 (16.5, 0) -> (4, 0)
  line L11 (4, 0) -> (4, 2)
  point P0 (13.5, 20.5)
  constraints: 16 end point, 4 parallel, 2 horizontal, 2 perpendicular
extrude "Extrusion57" add sketch "Sketch74" along normal blind 20 contours L9 L7 L11 L0 | L3 L4 L5 L0
sketch "Sketch75" plane through (65, -18.5, 3) normal (0, 1, 0) x (1, 0, 0)
  line L0 (-56, 16.5) -> (-56, 66) projected
  line L1 (0, 0) -> (-56, 0) projected
  line L2 (-56, 66) -> (-54, 66)
  line L3 (-54, 66) -> (-54, 0)
  line L4 (-54, 0) -> (-56, 0)
  line L5 (-56, 0) -> (-56, 66)
  point P0 (-65, 3)
  point P1 (-56, 0)
  dimension "d145" = 2
  constraints: 8 end point, 2 parallel, 1 horizontal, 1 perpendicular, 1 point on line
  measures "d145" distance of L3.end L4.end
extrude "Extrusion58" add sketch "Sketch75" along normal blind 2
sketch "Sketch76" plane through (82, 0, 0) normal (1, 0, 0) x (0, 0, -1)
  point P0 (0, 0)
sketch "Sketch77" plane through (82, 0, 0) normal (1, 0, 0) x (0, 0, -1)
  line L0 (2.0812, -18.5) -> (2.0812, -20.5) projected
  line L1 (2.0812, -20.5) -> (25.0812, -20.5) projected
  line L2 (2.0812, -18.5) -> (25.0812, -18.5)
  line L3 (25.0812, -18.5) -> (25.0812, -20.5)
  line L4 (25.0812, -20.5) -> (2.0812, -20.5)
  line L5 (2.0812, -20.5) -> (2.0812, -18.5)
  point P0 (0, 0)
  constraints: 8 end point, 2 parallel, 1 horizontal, 1 perpendicular
extrude "Extrusion59" cut sketch "Sketch77" against normal blind 2
sketch "Sketch78" plane through (65, -16.5, 3) normal (0, 1, 0) x (1, 0, 0)
  line L0 (-56, 12.5) -> (-56, 0) projected
  line L1 (-56, 66) -> (2, 66) projected
  line L2 (-56, 0) -> (-53.9374, 0)
  line L3 (-53.9374, 0) -> (-53.9374, 66)
  line L4 (-53.9374, 66) -> (-56, 66)
  line L5 (-56, 66) -> (-56, 0)
  point P0 (-65, 3)
  point P1 (-56, 12.5)
  constraints: 8 end point, 2 parallel, 1 horizontal, 1 perpendicular, 1 point on line
extrude "Extrusion60" add sketch "Sketch78" along normal blind 3
sketch "Sketch79" plane through (68, -18.5, -2.0812) normal (0, 1, 0) x (1, 0, 0)
  line L0 (14, -5.0812) -> (-1, -5.0812) projected
  line L1 (-1, 30.9188) -> (14, 30.9188) projected
  line L2 (14, -5.0812) -> (-0.0009, -5.0812)
  line L3 (-0.0009, -5.0812) -> (-0.0009, 30.9188)
  line L4 (-0.0009, 30.9188) -> (14, 30.9188)
  line L5 (14, 30.9188) -> (14, -5.0812)
  point P0 (-68, -2.0812)
  constraints: 8 end point, 2 parallel, 1 horizontal, 1 perpendicular, 1 point on line
extrude "Extrusion61" cut sketch "Sketch79" against normal blind 3
sketch "Sketch80" plane through (67.9991, -18.5, 3) normal (1, 0, 0) x (0, 0, -1)
  line L0 (0, 0) -> (0, 2) projected
  line L1 (36, -2) -> (66, -2) projected
  line L2 (0, 0) -> (36, 0)
  line L3 (36, 0) -> (36, -2)
  line L4 (36, -2) -> (0, -2)
  line L5 (0, -2) -> (0, 0)
  point P0 (3, 18.5)
  constraints: 8 end point, 2 parallel, 1 horizontal, 1 perpendicular
extrude "Extrusion62" add sketch "Sketch80" along normal blind 5
sketch "Sketch81" plane through (67, -18.5, 3) normal (0, 1, 0) x (1, 0, 0)
  point P0 (-67, 3)
sketch "Sketch82" plane through (29, 50, 3) normal (0, 0, 1) x (1, 0, 0)
  line L0 (38, -70.5) -> (43.9991, -70.5) projected
  line L1 (38, -68.5) -> (43.9991, -68.5) projected
  line L2 (43.9991, -70.5) -> (40.9991, -70.5)
  line L3 (40.9991, -70.5) -> (40.9991, -68.5)
  line L4 (40.9991, -68.5) -> (43.9991, -68.5)
  line L5 (43.9991, -68.5) -> (43.9991, -70.5)
  point P0 (-29, -50)
  dimension "d156" = 3
  constraints: 8 end point, 2 parallel, 1 horizontal, 1 perpendicular, 1 point on line
  measures "d156" distance of L3.end L4.end
extrude "Extrusion63" add sketch "Sketch82" along normal blind 10
sketch "Sketch83" plane through (72.9991, -18.5, 3) normal (1, 0, 0) x (0, 0, -1)
  line L0 (36, 0) -> (-10, 0) projected
  line L1 (36, -2) -> (-10, -2) projected
  line L2 (-10, 0) -> (-5, 0)
  line L3 (-5, 0) -> (-5, -2)
  line L4 (-5, -2) -> (-10, -2)
  line L5 (-10, -2) -> (-10, 0)
  point P0 (3, 18.5)
  point P1 (-5, 0)
  dimension "d159" = 5
  constraints: 8 end point, 2 parallel, 1 horizontal, 1 perpendicular, 1 point on line
  measures "d159" distance of L3.end L4.end
extrude "Extrusion64" add sketch "Sketch83" along normal blind 15.5
sketch "Sketch84" plane through (72.9991, -20.5, 8) normal (0, 0, -1) x (-1, 0, 0)
  line L0 (3, 2) -> (-15.5, 2) projected
  line L1 (0, 0) -> (-15.5, 0) projected
  line L2 (-15.5, 2) -> (-12.5, 2)
  line L3 (-12.5, 2) -> (-12.5, 0)
  line L4 (-12.5, 0) -> (-15.5, 0)
  line L5 (-15.5, 0) -> (-15.5, 2)
  point P0 (72.9991, 20.5)
  point P1 (-12.5, 2)
  dimension "d162" = 3
  constraints: 8 end point, 2 parallel, 1 horizontal, 1 perpendicular, 1 point on line
  measures "d162" distance of L3.end L4.end
extrude "Extrusion65" add sketch "Sketch84" along normal blind 26
sketch "Sketch85" plane through (85.4991, -20.5, 8) normal (-1, 0, 0) x (0, 0, 1)
  line L0 (-26, 2) -> (-26, 0) projected
  line L1 (-41, 0) -> (0, 0) projected
  line L2 (-26, 2) -> (-23, 2)
  line L3 (-23, 2) -> (-23, 0)
  line L4 (-23, 0) -> (-26, 0)
  line L5 (-26, 0) -> (-26, 2)
  point P0 (-8, 20.5)
  dimension "d165" = 3
  constraints: 8 end point, 2 parallel, 1 horizontal, 1 perpendicular, 1 point on line
  measures "d165" distance of L3.end L4.end
extrude "Extrusion66" add sketch "Sketch85" along normal up to surface (12.5 mm away)
sketch "Sketch86" plane through (72.9991, -20.5, -18) normal (0, 0, -1) x (-1, 0, 0)
  line L0 (-15.5, 2) -> (-15.5, 0) projected
  line L1 (63.9991, 0) -> (5.9991, 0) projected
  line L2 (-15.5, 2) -> (5.9991, 2)
  line L3 (5.9991, 2) -> (5.9991, 0)
  line L4 (5.9991, 0) -> (-15.5, 0)
  line L5 (-15.5, 0) -> (-15.5, 2)
  point P0 (72.9991, 20.5)
  constraints: 8 end point, 2 parallel, 1 horizontal, 1 perpendicular
extrude "Extrusion67" add sketch "Sketch86" along normal blind 10
sketch "Sketch87" plane through (67, -18.5, 3) normal (0, 1, 0) x (1, 0, 0)
  line L0 (5.9991, -5) -> (18.4991, -5) projected
  line L1 (18.4991, 18) -> (5.9991, 18) projected
  circle A0 centre (12.2491, -7) radius 1
  circle A1 centre (12.2491, 20) radius 1
  point P0 (-67, 3)
  point P1 (12.2491, -5)
  point P2 (12.2491, 18)
  dimension "d170" = 2
  dimension "d171" = 2
  constraints: 2 centre point, 2 midpoint
  measures "d170" diameter of A0
  measures "d171" diameter of A1
extrude "Extrusion68" cut sketch "Sketch87" against normal blind 10
thread "Thread3" size "M2x0.4" class "6H" standard "ANSI Metric M Profile" full length
thread "Thread4" size "M2x0.4" class "6H" standard "ANSI Metric M Profile" full length
sketch "Sketch88" plane through (2, 0, -33) normal (0, 0, -1) x (-1, 0, 0)
  line L0 (-70.9991, -18.5) -> (-70.9991, -20.5) projected
  line L1 (-65, -20.5) -> (-70.9991, -20.5) projected
  line L2 (-70.9991, -18.5) -> (-65, -18.5)
  line L3 (-65, -18.5) -> (-65, -20.5)
  line L4 (-65, -20.5) -> (-70.9991, -20.5)
  line L5 (-70.9991, -20.5) -> (-70.9991, -18.5)
  point P0 (2, 0)
  constraints: 8 end point, 2 parallel, 1 horizontal, 1 perpendicular
extrude "Extrusion69" cut sketch "Sketch88" against normal up to surface (5 mm away)
body "Solid1"
